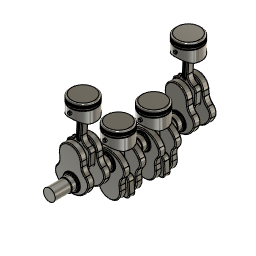
Piston&Crankshaft v11_neerav (Autodesk Fusion 360 design; units mm, degrees)
Autodesk Fusion 360 part; units mm, degrees
note: some values were not read from the file. Set by a fixed rule: which face or edge a step refers to.
sketch "Sketch1" plane through (0, 0, 0) normal (0, 1, 0) x (1, 0, 0) in component "piston"
  line L0 (0, 0) -> (40, 0)
  line L1 (40, 0) -> (40, -55)
  line L2 (40, -55) -> (0, -55)
  line L3 (0, -55) -> (0, 0)
  line L4 (40, -48) -> (36, -48)
  line L5 (36, -48) -> (36, -46)
  line L6 (36, -46) -> (40, -46)
  line L7 (40, -46) -> (40, -48)
  line L8 (40, -44) -> (36, -44)
  line L9 (36, -44) -> (36, -42)
  line L10 (36, -42) -> (40, -42)
  line L11 (40, -42) -> (40, -44)
  line L12 (40, -38) -> (36, -38)
  line L13 (36, -38) -> (36, -36)
  line L14 (36, -36) -> (40, -36)
  line L15 (40, -36) -> (40, -38)
  dimension "d1" = 40
  dimension "d2" = 55
  dimension "d3" = 2
  dimension "d4" = 4
  dimension "d5" = 7
  dimension "d6" = 2
  dimension "d7" = 4
  dimension "d8" = 2
  dimension "d9" = 2
  dimension "d10" = 4
  dimension "d11" = 4
  constraint horizontal L0
  constraint vertical L1
  constraint horizontal L2
  constraint vertical L3
  constraint coincident L0.start L3.end
  constraint horizontal L4
  constraint vertical L5
  constraint horizontal L6
  constraint vertical L7
  constraint coincident L1 L4.start
  constraint horizontal L8
  constraint vertical L9
  constraint horizontal L10
  constraint vertical L11
  constraint coincident L1 L8.start
  constraint horizontal L12
  constraint vertical L13
  constraint horizontal L14
  constraint vertical L15
  constraint coincident L1 L12.start
  measures "d1" distance of L0.start L0.end
  measures "d2" distance of L0.start L2.end
  measures "d3" distance of L4.end L5.end
  measures "d4" distance of L4.start L4.end
  measures "d5" distance of L2 L4
  measures "d6" distance of L8.end L9.end
  measures "d7" distance of L8.start L8.end
  measures "d8" distance of L6 L8
  measures "d9" distance of L12.end L13.end
  measures "d10" distance of L12.start L12.end
  measures "d11" distance of L10 L12
revolve "Revolve1" add sketch "Sketch1" angle 360 about axis through (0, 0, 55) along (0, 0, -1) contours L0 L1 L2 L3 L4 L5 L6 L8 L9 L10 L12 L13 L14 makes body 1 in component "piston"
sketch "Sketch2" plane through (0, 0, 0) normal (0, 0, -1) x (1, 0, 0) in component "piston"
  circle A0 centre (0, 0) radius 40
  circle A1 centre (0, 0) radius 35
  dimension "d13" = 70
  constraint concentric A0 A1
  measures "d13" diameter of A1
extrude "Extrude1" cut sketch "Sketch2" against normal blind 50 contours A1 bodies 1 in component "piston"
fillet "Fillet1" radius 5 1 edges at (-37.2931, -14.4646, 55) on bodies 1 in component "piston"
sketch "Sketch3" plane through (0, 0, 0) normal (0, 1, 0) x (1, 0, 0) in component "piston"
  line L0 (-40, 0) -> (40, 0)
  line L1 (-40, -36) -> (40, -36)
  line L2 (0, 0) -> (0, -10)
  spline S0 degree 5 poles (-35.5, 0) (-34.08, -0.7585) (-31.24, -2.2092) (-26.98, -4.1866) (-21.3, -6.419) (-14.2, -8.4906) (-7.1, -9.7789) (0, -10.2199) (7.1, -9.7789) (14.2, -8.4906) (21.3, -6.419) (26.98, -4.1866) (31.24, -2.2092) (34.08, -0.7585) (35.5, 0) knots 0 0 0 0 0 0 0.1 0.2 0.3 0.4 0.5 0.6 0.7 0.8 0.9 1 1 1 1 1 1
  circle A0 centre (0, -24) radius 5
  dimension "d18" = 10
  dimension "d19" = 10
  dimension "d20" = 4.5
  dimension "d21" = 4.5
  dimension "d22" = 24
  constraint coincident L2.start origin
  constraint perpendicular L0 L2
  constraint coincident L0 S0.start
  constraint coincident L0 S0.end
  measures "d18" distance of L2.start L2.end
  measures "d19" diameter of A0
  measures "d20" distance of L0.start S0.start
  measures "d21" distance of L0.end S0.end
  measures "d22" distance of L2.start A0.centre
extrude "Extrude2" cut sketch "Sketch3" along normal mid plane 90 bodies 1 in component "piston"
pattern_linear "00000000-0000-0000-0000-000000000000" [suppressed] in component "Pistons"
sketch "Sketch1 (2)" plane through (0, 0, 0) normal (0, 1, 0) x (1, 0, 0) in component "Connecting Rod"
  circle A0 centre (0, -40) radius 5
  circle A1 centre (0, -40) radius 8.5
  circle A2 centre (0, 85) radius 22.5
  line L0 (8.5, -40) -> (8.5, 35)
  line L1 (0, 85) -> (36, 85)
  line L2 (36, 85) -> (36, 60)
  line L3 (36, 60) -> (33.5, 60)
  arc A3 (33.5, 60) -> (8.5, 35) centre (33.5, 35) ccw
  line L4 (0, 85) -> (0, 50) construction
  arc A4 (-8.5, 35) -> (-33.5, 60) centre (-33.5, 35) ccw
  line L5 (-36, 60) -> (-33.5, 60)
  line L6 (-36, 85) -> (-36, 60)
  line L7 (0, 85) -> (-36, 85)
  line L8 (-8.5, -40) -> (-8.5, 35)
  line L9 (-36, 85) -> (36, 85)
  line L10 (36, 85) -> (36, 117.5)
  line L11 (36, 117.5) -> (-36, 117.5)
  line L12 (-36, 117.5) -> (-36, 85)
  circle A5 centre (0, -25) radius 4.75
  circle A6 centre (0, 47.5) radius 4.75
  line L13 (-4.75, -25) -> (-4.75, 47.5)
  line L14 (4.75, -25) -> (4.75, 47.5)
  dimension "d29" = 10
  dimension "d30" = 17
  dimension "d31" = 45
  dimension "d32" = 125
  dimension "d33" = 36
  dimension "d34" = 25
  dimension "d35" = 25
  dimension "d36" = 72
  dimension "d37" = 32.5
  dimension "d38" = 9.5
  dimension "d39" = 9.5
  dimension "d40" = 15
  dimension "d41" = 37.5
  constraint concentric A0 A1
  constraint coincident A1 L0.start
  constraint tangent A1 L0
  constraint vertical L0
  constraint coincident A2.centre L1.start
  constraint horizontal L1
  constraint perpendicular L1 L2
  constraint perpendicular L0 L3
  constraint tangent L3 A3
  constraint tangent L0 A3
  constraint perpendicular L1 L4
  constraint symmetric L0.start L4 L8.start
  constraint symmetric A2.centre L4 L1.start
  constraint symmetric L1.end L4 L6.start
  constraint symmetric L2.end L4 L5.start
  constraint symmetric L3.end L4 A4.end
  constraint symmetric L0.end L4 A4.start
  constraint symmetric A3 L4 A4
  constraint horizontal L9
  constraint vertical L10
  constraint horizontal L11
  constraint vertical L12
  constraint coincident A5 L13.start
  constraint coincident A6 L13.end
  constraint tangent A6 L13
  constraint parallel L8 L13
  constraint coincident A5 L14.start
  constraint coincident A6 L14.end
  constraint tangent A6 L14
  constraint parallel L0 L14
  measures "d29" diameter of A0
  measures "d30" diameter of A1
  measures "d31" diameter of A2
  measures "d32" distance of A0.centre A2.centre
  measures "d33" distance of A2.centre L1.end
  measures "d34" distance of L1.end L2.end
  measures "d35" radius of A3
  measures "d36" distance of L6.start L1.end
  measures "d37" distance of L6.start L11.end
  measures "d38" diameter of A5
  measures "d39" diameter of A6
  measures "d40" distance of A0.centre A5.centre
  measures "d41" distance of A2.centre A6.centre
extrude "Extrude1'" add sketch "Sketch1 (2)" along normal mid plane 20 separate body contours A1 | A1 A2 L0 L1 L2 L3 A3 A4 L5 L6 L7 L8 L9 | A2 L1 L7 L9 L10 L11 L12 makes body 2 in component "Connecting Rod"
extrude "Extrude2'" add sketch "Sketch1 (2)" along normal mid plane 10 contours A5 | A5 A6 L13 L14 | A6 bodies 2 in component "Connecting Rod"
fillet "Fillet1'" radius 12.5 4 edges at (-36, 0, -60) (-36, 0, -117.5) (36, 0, -60) (36, 0, -117.5) on bodies 2 in component "Connecting Rod"
fillet "Fillet2" radius 2.5 24 edges at (-33.4478, -10, -63.573) (-36, -10, -88.071) (-32.3388, -10, -113.8388) (0, -10, -117.5) (32.3388, -10, -113.8388) (36, -10, -88.071) (33.4478, -10, -63.573) (13.6044, -10, -50.1383) (8.5, -10, 2.5) (0, -10, 48.5) (-8.5, -10, 2.5) (-13.6044, -10, -50.1383) (8.5, 10, 2.5) (13.6044, 10, -50.1383) (33.4478, 10, -63.573) (36, 10, -88.071) (32.3388, 10, -113.8388) (0, 10, -117.5) (-32.3388, 10, -113.8388) (-36, 10, -88.071) (-33.4478, 10, -63.573) (-13.6044, 10, -50.1383) (-8.5, 10, 2.5) (0, 10, 48.5) on bodies 2 in component "Connecting Rod"
fillet "Fillet3" radius 1.5 16 edges at (0, -5, 29.75) (4.75, -5, -11.25) (0, -5, -52.25) (-4.75, -5, -11.25) (0, -10, 29.75) (4.75, -10, -11.25) (0, -10, -52.25) (-4.75, -10, -11.25) (0, 10, 29.75) (-4.75, 10, -11.25) (0, 10, -52.25) (4.75, 10, -11.25) (4.75, 5, -11.25) (0, 5, 29.75) (-4.75, 5, -11.25) (0, 5, -52.25) on bodies 2 in component "Connecting Rod"
pattern_linear "00000000-0000-0000-0000-000000000000'" [suppressed] in component "Connecting Rods"
sketch "Sketch1 (3)" plane through (0, 0, 0) normal (0, 1, 0) x (1, 0, 0) in component "Pin"
cylinder "CylinderPrimitive1" add diameter 10 height 90 placed x (1, 0, 0) y (0, 0, -1) z (0, 1, 0) at (50, 0, 40) separate body makes body 3 in component "Pin"
fillet "Fillet1''" radius 1.5 2 edges at (45.3384, 0, 38.1919) (45.3384, 90, 41.8081) on bodies 3 in component "Pin"
pattern_linear "00000000-0000-0000-0000-000000000000''" [suppressed] in component "Pins"
sketch "Sketch1 (4)" plane through (0, 0, 0) normal (0, 1, 0) x (1, 0, 0) in component "Crankshaft"
  circle A0 centre (0, 85) radius 22.5
  circle A1 centre (0, 85) radius 35
  circle A2 centre (0, 20.5) radius 20
  circle A3 centre (0, 20.5) radius 25
  arc A4 (-55, 42.5) -> (55, 42.5) centre (0, 42.5) ccw
  line L0 (-35, 85) -> (-35, 42.5)
  line L1 (35, 85) -> (35, 42.5)
  line L2 (-35, 42.5) -> (-55, 42.5)
  line L3 (35, 42.5) -> (55, 42.5)
  dimension "d64" = 70
  dimension "d66" = 40
  dimension "d67" = 50
  dimension "d68" = 42.5
  dimension "d69" = 22
  constraint concentric A0 A1
  constraint concentric A2 A3
  constraint coincident A1 L0.start
  constraint tangent A1 L0
  constraint coincident A1 L1.start
  constraint tangent A1 L1
  measures "d64" diameter of A1
  measures "d66" diameter of A2
  measures "d67" diameter of A3
  measures "d68" distance of A0.centre A4.centre
  measures "d69" distance of A2.centre A4.centre
extrude "Extrude1''" add sketch "Sketch1 (4)" along normal blind 20 from surface at 15 separate body contours A0 | A1 | A1 A4 L0 L1 L2 L3 | A2 | A3 makes body 4 in component "Crankshaft"
extrude "Extrude2''" add sketch "Sketch1 (4)" along normal blind 20 from surface at 35 contours A2 bodies 4 in component "Crankshaft"
extrude "Extrude3" add sketch "Sketch1 (4)" along normal blind 5 from surface at 35 contours A3 bodies 4 in component "Crankshaft"
fillet "Fillet1'''" radius 30 2 edges at (35, 25, -42.5) (-35, 25, -42.5) on bodies 4 in component "Crankshaft"
fillet "Fillet2'" radius 25 2 edges at (55, 25, -42.5) (-55, 25, -42.5) on bodies 4 in component "Crankshaft"
fillet "Fillet3'" radius 2.5 16 edges at (51.987, 35, -35.6375) (37.4915, 35, -58.8142) (35, 35, -77.8921) (0, 35, -120) (-35, 35, -77.8921) (-37.4915, 35, -58.8142) (-51.987, 35, -35.6375) (0, 35, 12.5) (37.4915, 15, -58.8142) (35, 15, -77.8921) (0, 15, -120) (-35, 15, -77.8921) (-37.4915, 15, -58.8142) (-51.987, 15, -35.6375) (0, 15, 12.5) (51.987, 15, -35.6375) on bodies 4 in component "Crankshaft"
fillet "Fillet4" radius 1.5 3 edges at (-18.6465, 55, -13.2677) (-23.3082, 40, -11.4596) (-23.3082, 35, -29.5404) on bodies 4 in component "Crankshaft"
mirror "Mirror1" about plane through (0, 0, 0) normal (0, 1, 0) of bodies 4 makes body 5 in component "Crankshaft"
extrude "Extrude4" add sketch "Sketch1 (4)" along normal mid plane 30 contours A0 bodies 4 5 in component "Crankshaft"
pattern_linear "R-Pattern1" count 4 spacing 110 along (0, -1, 0) of bodies 4 makes body 6 at (-26.5501, -95, -38.8431) makes body 7 at (-26.5501, -205, -38.8431) makes body 8 at (-26.5501, -315, -38.8431) in component "Crankshaft"
move_body "Move1" bodies 7 6 to x (-1, 0, 0) y (0, 1, 0) z (0, 0, -1) at (0, 0, -41) in component "Crankshaft"
combine "Combine1" operation add target body 8 tool bodies 7 4 6 in component "Crankshaft"
extrude "Extrude5" add 1 faces at (1.2503, -385, -15.2969) along direction (0, -1, 0) blind 50 on bodies 8 bodies 8 in component "Crankshaft"
sketch "Sketch1 (5)" plane through (0, -435, 0) normal (0, -1, 0) x (1, 0, 0)
  circle A0 centre (0, -20.5) radius 18.5
  circle A1 centre (0, -20.5) radius 37.5
  dimension "d97" = 75
  constraint concentric A0 A1
  measures "d97" diameter of A1
extrude "Extrude1'''" add sketch "Sketch1 (5)" against normal blind 20 separate body makes body 9 in component "Component"
sketch "Sketch2 (2)" plane through (0, 0, 200) normal (0, 0, 1) x (-1, 0, 0)
  circle A0 centre (0, 114.9976) radius 35
  line L0 (-138.5511, 475.8344) -> (152.1462, 475.8344)
  line L1 (152.1462, 475.8344) -> (152.1462, -88.8296)
  line L2 (152.1462, -88.8296) -> (-138.5511, -88.8296)
  line L3 (-138.5511, -88.8296) -> (-138.5511, 475.8344)
  circle A1 centre (0, 6.5024) radius 40
  circle A2 centre (0, 114.9976) radius 40
  circle A3 centre (0, 224.9976) radius 40
  circle A4 centre (0, 334.9976) radius 40
  constraint horizontal L0
  constraint vertical L1
  constraint horizontal L2
  constraint vertical L3
extrude "Extrude1''''" add sketch "Sketch2 (2)" along normal blind 25 separate body contours L0 L1 L2 L3 makes body 10 in component "Component'"
component "Pistons" placed x (1, 0, 0) y (0, 1, 0) z (0, 0, 1) at (0, 0, 0)
component "Connecting Rods" placed x (1, 0, 0) y (0, 1, 0) z (0, 0, 1) at (0, 0, 0)
component "Pins" placed x (1, 0, 0) y (0, 1, 0) z (0, 0, 1) at (0, 0, 0)
component "Crankshaft" placed x (-1, 0, 0) y (0, 1, 0) z (0, 0, -1) at (0, -5, -41)
component "Component" placed x (1, 0, 0) y (0, 1, 0) z (0, 0, 1) at (0, 0, 0)
component "Component'" placed x (1, 0, 0) y (0, 1, 0) z (0, 0, 1) at (0, 0, 0)
component "piston" placed x (1, 0, 0) y (0, 1, 0) z (0, 0, 1) at (0, -6.5024, 145) in component "Pistons"
component "piston" placed x (1, 0, 0) y (0, 1, 0) z (0, 0, 1) at (0, -114.9976, 16) in component "Pistons"
component "piston" placed x (1, 0, 0) y (0, 1, 0) z (0, 0, 1) at (0, -224.9976, 16) in component "Pistons"
component "piston" placed x (1, 0, 0) y (0, 1, 0) z (0, 0, 1) at (0, -334.9976, 145) in component "Pistons"
component "Connecting Rod" placed x (1, 0, 0) y (0, 1, 0) z (0, 0, 1) at (0, -5, 129) in component "Connecting Rods"
component "Connecting Rod" placed x (1, 0, 0) y (0, 1, 0) z (0, 0, 1) at (0, -115, 0) in component "Connecting Rods"
component "Connecting Rod" placed x (1, 0, 0) y (0, 1, 0) z (0, 0, 1) at (0, -225, 0) in component "Connecting Rods"
component "Connecting Rod" placed x (1, 0, 0) y (0, 1, 0) z (0, 0, 1) at (0, -335, 129) in component "Connecting Rods"
component "Pin" placed x (1, 0, 0) y (0, 1, 0) z (0, 0, 1) at (-50, -50, 129) in component "Pins"
component "Pin" placed x (1, 0, 0) y (0, 1, 0) z (0, 0, 1) at (-50, -160, 0) in component "Pins"
component "Pin" placed x (1, 0, 0) y (0, 1, 0) z (0, 0, 1) at (-50, -270, 0) in component "Pins"
component "Pin" placed x (1, 0, 0) y (0, 1, 0) z (0, 0, 1) at (-50, -380, 129) in component "Pins"
